Autodesk Inventor part; units mm, degrees
(part 3 of 3)
  arc A872 (130.3995, -26.0356) -> (130.7044, -25.7308) centre (130.3995, -25.7308) ccw
  line L653 (130.3995, -11.9894) -> (116.9629, -11.9894)
  arc A873 (90.4644, -25.7308) -> (90.7692, -26.0356) centre (90.7692, -25.7308) ccw
  arc A874 (90.7692, -11.9894) -> (90.4644, -12.2942) centre (90.7692, -12.2942) ccw
  line L654 (90.4644, -12.2942) -> (90.4644, -25.7308)
  arc A875 (104.5106, -12.2942) -> (104.2058, -11.9894) centre (104.2058, -12.2942) ccw
  line L655 (104.5106, -25.7308) -> (104.5106, -12.2942)
  line L656 (90.7692, -26.0356) -> (104.2058, -26.0356)
  line L657 (90.4644, -26.0356) -> (104.5106, -11.9894) construction
  line L658 (104.5106, -26.0356) -> (90.4644, -11.9894) construction
  arc A876 (104.2058, -26.0356) -> (104.5106, -25.7308) centre (104.2058, -25.7308) ccw
  line L659 (104.2058, -11.9894) -> (90.7692, -11.9894)
  arc A877 (135.7082, -6.6808) -> (136.0129, -6.9856) centre (136.0129, -6.6808) ccw
  arc A878 (136.0129, 7.0606) -> (135.7082, 6.7558) centre (136.0129, 6.7558) ccw
  line L660 (135.7082, 6.7558) -> (135.7082, -6.6808)
  arc A879 (149.7544, 6.7558) -> (149.4495, 7.0606) centre (149.4495, 6.7558) ccw
  line L661 (149.7544, -6.6808) -> (149.7544, 6.7558)
  line L662 (136.0129, -6.9856) -> (149.4495, -6.9856)
  line L663 (135.7082, -6.9856) -> (149.7544, 7.0606) construction
  line L664 (149.7544, -6.9856) -> (135.7082, 7.0606) construction
  arc A880 (149.4495, -6.9856) -> (149.7544, -6.6808) centre (149.4495, -6.6808) ccw
  line L665 (149.4495, 7.0606) -> (136.0129, 7.0606)
  arc A881 (135.7082, 12.3692) -> (136.0129, 12.0644) centre (136.0129, 12.3692) ccw
  arc A882 (136.0129, 26.1106) -> (135.7082, 25.8058) centre (136.0129, 25.8058) ccw
  line L666 (135.7082, 25.8058) -> (135.7082, 12.3692)
  arc A883 (149.7544, 25.8058) -> (149.4495, 26.1106) centre (149.4495, 25.8058) ccw
  line L667 (149.7544, 12.3692) -> (149.7544, 25.8058)
  line L668 (136.0129, 12.0644) -> (149.4495, 12.0644)
  line L669 (135.7082, 12.0644) -> (149.7544, 26.1106) construction
  line L670 (149.7544, 12.0644) -> (135.7082, 26.1106) construction
  arc A884 (149.4495, 12.0644) -> (149.7544, 12.3692) centre (149.4495, 12.3692) ccw
  line L671 (149.4495, 26.1106) -> (136.0129, 26.1106)
  arc A885 (135.7082, 31.4192) -> (136.0129, 31.1144) centre (136.0129, 31.4192) ccw
  arc A886 (136.0129, 45.1606) -> (135.7082, 44.8558) centre (136.0129, 44.8558) ccw
  line L672 (135.7082, 44.8558) -> (135.7082, 31.4192)
  arc A887 (149.7544, 44.8558) -> (149.4495, 45.1606) centre (149.4495, 44.8558) ccw
  line L673 (149.7544, 31.4192) -> (149.7544, 44.8558)
  line L674 (136.0129, 31.1144) -> (149.4495, 31.1144)
  line L675 (135.7082, 31.1144) -> (149.7544, 45.1606) construction
  line L676 (149.7544, 31.1144) -> (135.7082, 45.1606) construction
  arc A888 (149.4495, 31.1144) -> (149.7544, 31.4192) centre (149.4495, 31.4192) ccw
  line L677 (149.4495, 45.1606) -> (136.0129, 45.1606)
  arc A889 (78.5582, 31.4192) -> (78.863, 31.1144) centre (78.863, 31.4192) ccw
  arc A890 (78.863, 45.1606) -> (78.5582, 44.8558) centre (78.863, 44.8558) ccw
  line L678 (78.5582, 44.8558) -> (78.5582, 31.4192)
  arc A891 (92.6044, 44.8558) -> (92.2996, 45.1606) centre (92.2996, 44.8558) ccw
  line L679 (92.6044, 31.4192) -> (92.6044, 44.8558)
  line L680 (78.863, 31.1144) -> (92.2996, 31.1144)
  line L681 (78.5582, 31.1144) -> (92.6044, 45.1606) construction
  line L682 (92.6044, 31.1144) -> (78.5582, 45.1606) construction
  arc A892 (92.2996, 31.1144) -> (92.6044, 31.4192) centre (92.2996, 31.4192) ccw
  line L683 (92.2996, 45.1606) -> (78.863, 45.1606)
  arc A893 (88.0832, 12.3692) -> (88.388, 12.0644) centre (88.388, 12.3692) ccw
  arc A894 (88.388, 26.1106) -> (88.0832, 25.8058) centre (88.388, 25.8058) ccw
  line L684 (88.0832, 25.8058) -> (88.0832, 12.3692)
  arc A895 (102.1294, 25.8058) -> (101.8246, 26.1106) centre (101.8246, 25.8058) ccw
  line L685 (102.1294, 12.3692) -> (102.1294, 25.8058)
  line L686 (88.388, 12.0644) -> (101.8246, 12.0644)
  line L687 (88.0832, 12.0644) -> (102.1294, 26.1106) construction
  line L688 (102.1294, 12.0644) -> (88.0832, 26.1106) construction
  arc A896 (101.8246, 12.0644) -> (102.1294, 12.3692) centre (101.8246, 12.3692) ccw
  line L689 (101.8246, 26.1106) -> (88.388, 26.1106)
  arc A897 (111.8957, 12.3692) -> (112.2004, 12.0644) centre (112.2004, 12.3692) ccw
  arc A898 (112.2004, 26.1106) -> (111.8957, 25.8058) centre (112.2004, 25.8058) ccw
  line L690 (111.8957, 25.8058) -> (111.8957, 12.3692)
  arc A899 (125.9419, 25.8058) -> (125.6371, 26.1106) centre (125.6371, 25.8058) ccw
  line L691 (125.9419, 12.3692) -> (125.9419, 25.8058)
  line L692 (112.2004, 12.0644) -> (125.6371, 12.0644)
  line L693 (111.8957, 12.0644) -> (125.9419, 26.1106) construction
  line L694 (125.9419, 12.0644) -> (111.8957, 26.1106) construction
  arc A900 (125.6371, 12.0644) -> (125.9419, 12.3692) centre (125.6371, 12.3692) ccw
  line L695 (125.6371, 26.1106) -> (112.2004, 26.1106)
  line L696 (-138.1229, -13.7293) -> (-122.5019, -13.7293)
  line L697 (-144.6761, -26.4293) -> (-141.5265, -26.4293)
  line L698 (-141.5265, -25.2101) -> (-139.7231, -25.2101)
  line L699 (-144.6761, -25.2101) -> (-144.6761, -26.4293)
  line L700 (-146.4795, -19.0125) -> (-146.4795, -25.2101)
  line L701 (-139.7231, -24.3211) -> (-139.7231, -13.7293)
  line L702 (-146.4795, -25.2101) -> (-144.6761, -25.2101)
  line L703 (-146.4795, -12.8149) -> (-139.7231, -12.8149)
  line L704 (-139.7231, -12.8149) -> (-146.4795, -25.2101) construction
  line L705 (-146.4795, -12.8149) -> (-139.7231, -25.2101) construction
  line L706 (-139.7231, -25.2101) -> (-139.7231, -24.3211)
  line L707 (-147.4193, -16.0153) -> (-147.4193, -19.0125)
  line L708 (-147.4193, -19.0125) -> (-146.4795, -19.0125)
  line L709 (-146.4795, -16.0153) -> (-147.4193, -16.0153)
  line L710 (-146.4795, -12.8149) -> (-146.4795, -16.0153)
  line L711 (-120.6985, -26.4293) -> (-120.6985, -25.2101)
  line L712 (-120.6985, -25.2101) -> (-122.5019, -25.2101)
  line L713 (-117.5489, -26.4293) -> (-120.6985, -26.4293)
  line L714 (-122.5019, -25.2101) -> (-122.5019, -24.3211)
  line L715 (-141.5265, -26.4293) -> (-141.5265, -25.2101)
  circle A901 centre (-143.0505, -27.2675) radius 1.994
  line L716 (-139.7231, -24.3211) -> (-138.1229, -24.3211)
  circle A902 centre (-119.1745, -27.2675) radius 1.994
  line L717 (-115.7455, -25.2101) -> (-117.5489, -25.2101)
  line L718 (-143.1013, -12.8149) -> (-143.1013, -26.4293)
  line L719 (-117.5489, -25.2101) -> (-117.5489, -26.4293)
  circle A903 centre (-119.1745, -12.0275) radius 1.524
  circle A904 centre (-143.0505, -12.0275) radius 1.524
  line L720 (-138.1229, -24.3211) -> (-122.5019, -24.3211)
  line L721 (-139.7231, -12.8149) -> (-139.7231, -13.7293)
  line L722 (-139.7231, -13.7293) -> (-138.1229, -13.7293)
  arc A905 (-137.8181, -12.0021) -> (-138.1229, -12.3069) centre (-137.8181, -12.3069) ccw
  line L723 (-131.1125, -19.0125) -> (-143.1013, -19.0125)
  line L724 (-131.1125, -12.0021) -> (-131.1125, -26.0229)
  line L725 (-124.1021, -12.0021) -> (-138.1229, -26.0229) construction
  arc A906 (-124.1021, -12.3069) -> (-124.4069, -12.0021) centre (-124.4069, -12.3069) ccw
  arc A907 (-138.1229, -25.7181) -> (-137.8181, -26.0229) centre (-137.8181, -25.7181) ccw
  line L726 (-138.1229, -25.7181) -> (-138.1229, -12.3069)
  line L727 (-124.4069, -26.0229) -> (-137.8181, -26.0229)
  line L728 (-138.1229, -12.0021) -> (-124.1021, -26.0229) construction
  line L729 (-137.8181, -12.0021) -> (-124.4069, -12.0021)
  line L730 (-119.1237, -12.8149) -> (-119.1237, -26.4293)
  line L731 (-115.7455, -19.0125) -> (-115.7455, -25.2101)
  line L732 (-115.7455, -12.8149) -> (-115.7455, -16.0153)
  line L733 (-115.7455, -16.0153) -> (-114.8057, -16.0153)
  line L734 (-114.8057, -16.0153) -> (-114.8057, -19.0125)
  arc A908 (-124.4069, -26.0229) -> (-124.1021, -25.7181) centre (-124.4069, -25.7181) ccw
  line L735 (-124.1021, -12.3069) -> (-124.1021, -25.7181)
  line L736 (-122.5019, -24.3211) -> (-122.5019, -13.7293)
  line L737 (-122.5019, -12.8149) -> (-122.5019, -13.7293)
  line L738 (-131.1125, -19.0125) -> (-119.1237, -19.0125)
  line L739 (-114.8057, -19.0125) -> (-115.7455, -19.0125)
  line L740 (-115.7455, -12.8149) -> (-122.5019, -12.8149)
  line L741 (-115.7455, -12.8149) -> (-122.5019, -25.2101) construction
  line L742 (-122.5019, -12.8149) -> (-115.7455, -25.2101) construction
  line L743 (107.1458, 43.4207) -> (122.7669, 43.4207)
  line L744 (100.5926, 30.7207) -> (103.7422, 30.7207)
  line L745 (103.7422, 31.9399) -> (105.5456, 31.9399)
  line L746 (100.5926, 31.9399) -> (100.5926, 30.7207)
  line L747 (98.7892, 38.1375) -> (98.7892, 31.9399)
  line L748 (105.5456, 32.8289) -> (105.5456, 43.4207)
  line L749 (98.7892, 31.9399) -> (100.5926, 31.9399)
  line L750 (98.7892, 44.3351) -> (105.5456, 44.3351)
  line L751 (105.5456, 44.3351) -> (98.7892, 31.9399) construction
  line L752 (98.7892, 44.3351) -> (105.5456, 31.9399) construction
  line L753 (105.5456, 31.9399) -> (105.5456, 32.8289)
  line L754 (97.8495, 41.1347) -> (97.8495, 38.1375)
  line L755 (97.8495, 38.1375) -> (98.7892, 38.1375)
  line L756 (98.7892, 41.1347) -> (97.8495, 41.1347)
  line L757 (98.7892, 44.3351) -> (98.7892, 41.1347)
  line L758 (124.5702, 30.7207) -> (124.5702, 31.9399)
  line L759 (124.5702, 31.9399) -> (122.7669, 31.9399)
  line L760 (127.7198, 30.7207) -> (124.5702, 30.7207)
  line L761 (122.7669, 31.9399) -> (122.7669, 32.8289)
  line L762 (103.7422, 30.7207) -> (103.7422, 31.9399)
  circle A909 centre (102.2182, 29.8825) radius 1.994
  line L763 (105.5456, 32.8289) -> (107.1458, 32.8289)
  circle A910 centre (126.0942, 29.8825) radius 1.994
  line L764 (129.5232, 31.9399) -> (127.7198, 31.9399)
  line L765 (102.1675, 44.3351) -> (102.1675, 30.7207)
  line L766 (127.7198, 31.9399) -> (127.7198, 30.7207)
  circle A911 centre (126.0942, 45.1225) radius 1.524
  circle A912 centre (102.2182, 45.1225) radius 1.524
  line L767 (107.1458, 32.8289) -> (122.7669, 32.8289)
  line L768 (105.5456, 44.3351) -> (105.5456, 43.4207)
  line L769 (105.5456, 43.4207) -> (107.1458, 43.4207)
  arc A913 (107.4506, 45.1479) -> (107.1458, 44.8431) centre (107.4506, 44.8431) ccw
  line L770 (114.1562, 38.1375) -> (102.1675, 38.1375)
  line L771 (114.1562, 45.1479) -> (114.1562, 31.1271)
  line L772 (121.1666, 45.1479) -> (107.1458, 31.1271) construction
  arc A914 (121.1666, 44.8431) -> (120.8618, 45.1479) centre (120.8618, 44.8431) ccw
  arc A915 (107.1458, 31.4319) -> (107.4506, 31.1271) centre (107.4506, 31.4319) ccw
  line L773 (107.1458, 31.4319) -> (107.1458, 44.8431)
  line L774 (120.8618, 31.1271) -> (107.4506, 31.1271)
  line L775 (107.1458, 45.1479) -> (121.1666, 31.1271) construction
  line L776 (107.4506, 45.1479) -> (120.8618, 45.1479)
  line L777 (126.145, 44.3351) -> (126.145, 30.7207)
  line L778 (129.5232, 38.1375) -> (129.5232, 31.9399)
  line L779 (129.5232, 44.3351) -> (129.5232, 41.1347)
  line L780 (129.5232, 41.1347) -> (130.463, 41.1347)
  line L781 (130.463, 41.1347) -> (130.463, 38.1375)
  arc A916 (120.8618, 31.1271) -> (121.1666, 31.4319) centre (120.8618, 31.4319) ccw
  line L782 (121.1666, 44.8431) -> (121.1666, 31.4319)
  line L783 (122.7669, 32.8289) -> (122.7669, 43.4207)
  line L784 (122.7669, 44.3351) -> (122.7669, 43.4207)
  line L785 (114.1562, 38.1375) -> (126.145, 38.1375)
  line L786 (130.463, 38.1375) -> (129.5232, 38.1375)
  line L787 (129.5232, 44.3351) -> (122.7669, 44.3351)
  line L788 (129.5232, 44.3351) -> (122.7669, 31.9399) construction
  line L789 (122.7669, 44.3351) -> (129.5232, 31.9399) construction
  line L790 (104.7646, 5.3207) -> (120.3856, 5.3207)
  line L791 (98.2114, -7.3793) -> (101.361, -7.3793)
  line L792 (101.361, -6.1601) -> (103.1644, -6.1601)
  line L793 (98.2114, -6.1601) -> (98.2114, -7.3793)
  line L794 (96.408, 0.0375) -> (96.408, -6.1601)
  line L795 (103.1644, -5.2711) -> (103.1644, 5.3207)
  line L796 (96.408, -6.1601) -> (98.2114, -6.1601)
  line L797 (96.408, 6.2351) -> (103.1644, 6.2351)
  line L798 (103.1644, 6.2351) -> (96.408, -6.1601) construction
  line L799 (96.408, 6.2351) -> (103.1644, -6.1601) construction
  line L800 (103.1644, -6.1601) -> (103.1644, -5.2711)
  line L801 (95.4682, 3.0347) -> (95.4682, 0.0375)
  line L802 (95.4682, 0.0375) -> (96.408, 0.0375)
  line L803 (96.408, 3.0347) -> (95.4682, 3.0347)
  line L804 (96.408, 6.2351) -> (96.408, 3.0347)
  line L805 (122.189, -7.3793) -> (122.189, -6.1601)
  line L806 (122.189, -6.1601) -> (120.3856, -6.1601)
  line L807 (125.3386, -7.3793) -> (122.189, -7.3793)
  line L808 (120.3856, -6.1601) -> (120.3856, -5.2711)
  line L809 (101.361, -7.3793) -> (101.361, -6.1601)
  circle A917 centre (99.837, -8.2175) radius 1.994
  line L810 (103.1644, -5.2711) -> (104.7646, -5.2711)
  circle A918 centre (123.713, -8.2175) radius 1.994
  line L811 (127.142, -6.1601) -> (125.3386, -6.1601)
  line L812 (99.7862, 6.2351) -> (99.7862, -7.3793)
  line L813 (125.3386, -6.1601) -> (125.3386, -7.3793)
  circle A919 centre (123.713, 7.0225) radius 1.524
  circle A920 centre (99.837, 7.0225) radius 1.524
  line L814 (104.7646, -5.2711) -> (120.3856, -5.2711)
  line L815 (103.1644, 6.2351) -> (103.1644, 5.3207)
  line L816 (103.1644, 5.3207) -> (104.7646, 5.3207)
  arc A921 (105.0694, 7.0479) -> (104.7646, 6.7431) centre (105.0694, 6.7431) ccw
  line L817 (111.775, 0.0375) -> (99.7862, 0.0375)
  line L818 (111.775, 7.0479) -> (111.775, -6.9729)
  line L819 (118.7854, 7.0479) -> (104.7646, -6.9729) construction
  arc A922 (118.7854, 6.7431) -> (118.4806, 7.0479) centre (118.4806, 6.7431) ccw
  arc A923 (104.7646, -6.6681) -> (105.0694, -6.9729) centre (105.0694, -6.6681) ccw
  line L820 (104.7646, -6.6681) -> (104.7646, 6.7431)
  line L821 (118.4806, -6.9729) -> (105.0694, -6.9729)
  line L822 (104.7646, 7.0479) -> (118.7854, -6.9729) construction
  line L823 (105.0694, 7.0479) -> (118.4806, 7.0479)
  line L824 (123.7638, 6.2351) -> (123.7638, -7.3793)
  line L825 (127.142, 0.0375) -> (127.142, -6.1601)
  line L826 (127.142, 6.2351) -> (127.142, 3.0347)
  line L827 (127.142, 3.0347) -> (128.0818, 3.0347)
  line L828 (128.0818, 3.0347) -> (128.0818, 0.0375)
  arc A924 (118.4806, -6.9729) -> (118.7854, -6.6681) centre (118.4806, -6.6681) ccw
  line L829 (118.7854, 6.7431) -> (118.7854, -6.6681)
  line L830 (120.3856, -5.2711) -> (120.3856, 5.3207)
  line L831 (120.3856, 6.2351) -> (120.3856, 5.3207)
  line L832 (111.775, 0.0375) -> (123.7638, 0.0375)
  line L833 (128.0818, 0.0375) -> (127.142, 0.0375)
  line L834 (127.142, 6.2351) -> (120.3856, 6.2351)
  line L835 (127.142, 6.2351) -> (120.3856, -6.1601) construction
  line L836 (120.3856, 6.2351) -> (127.142, -6.1601) construction
  circle A925 centre (-71.613, -46.3175) radius 1.994
  circle A926 centre (28.463, -31.0775) radius 1.524
  circle A927 centre (28.463, -46.3175) radius 1.994
  circle A928 centre (-71.613, -31.0775) radius 1.524
  line L837 (31.8031, -31.8649) -> (31.8031, -35.0653)
  line L838 (31.8031, -44.2601) -> (29.9997, -44.2601)
  line L839 (29.9997, -44.2601) -> (29.9997, -45.4793)
  line L840 (26.8501, -45.4793) -> (26.8501, -44.2601)
  line L841 (26.8501, -44.2601) -> (25.0467, -44.2601)
  line L842 (25.0467, -44.2601) -> (25.0467, -43.3711)
  line L843 (25.0467, -31.8649) -> (25.0467, -32.7793)
  line L844 (25.0467, -43.3711) -> (25.0467, -32.7793)
  line L845 (29.9997, -45.4793) -> (26.8501, -45.4793)
  line L846 (28.4249, -31.8649) -> (28.4249, -45.4793)
  line L847 (31.8031, -38.0625) -> (31.8031, -44.2601)
  line L848 (32.7429, -38.0625) -> (31.8031, -38.0625)
  line L849 (25.0467, -31.8649) -> (31.8031, -44.2601) construction
  line L850 (31.8031, -35.0653) -> (32.7429, -35.0653)
  line L851 (32.7429, -35.0653) -> (32.7429, -38.0625)
  line L852 (31.8031, -31.8649) -> (25.0467, -44.2601) construction
  line L853 (31.8031, -31.8649) -> (25.0467, -31.8649)
  arc A929 (-14.8694, -45.0729) -> (-14.5646, -44.7681) centre (-14.8694, -44.7681) ccw
  line L854 (25.0467, -35.8125) -> (-21.575, -35.8125)
  line L855 (-21.575, -38.0625) -> (28.4249, -38.0625)
  line L856 (25.0467, -40.3125) -> (-21.575, -40.3125)
  line L857 (-71.5749, -31.8649) -> (-71.5749, -45.4793)
  line L858 (-75.8929, -38.0625) -> (-74.9531, -38.0625)
  line L859 (-64.9489, -38.0625) -> (-64.9489, -35.8125)
  line L860 (-68.1967, -35.8125) -> (-21.575, -35.8125)
  line L861 (-21.575, -38.0625) -> (-71.5749, -38.0625)
  line L862 (-68.1967, -40.3125) -> (-21.575, -40.3125)
  arc A930 (-28.2806, -31.0521) -> (-28.5854, -31.3569) centre (-28.2806, -31.3569) ccw
  arc A931 (-28.5854, -44.7681) -> (-28.2806, -45.0729) centre (-28.2806, -44.7681) ccw
  line L863 (-28.5854, -31.3569) -> (-28.5854, -44.7681)
  line L864 (-14.8694, -31.0521) -> (-28.2806, -31.0521)
  line L865 (-28.5854, -45.0729) -> (-14.5646, -31.0521) construction
  line L866 (-14.5646, -45.0729) -> (-28.5854, -31.0521) construction
  line L867 (-14.5646, -44.7681) -> (-14.5646, -31.3569)
  line L868 (-21.575, -31.0521) -> (-21.575, -45.0729)
  line L869 (-28.2806, -45.0729) -> (-14.8694, -45.0729)
  line L870 (-74.9531, -35.0653) -> (-75.8929, -35.0653)
  arc A932 (-14.5646, -31.3569) -> (-14.8694, -31.0521) centre (-14.8694, -31.3569) ccw
  line L871 (-62.9931, -38.0625) -> (-62.9931, -40.3125)
  line L872 (-68.1967, -43.3711) -> (-68.1967, -32.7793)
  line L873 (-70.0001, -45.4793) -> (-70.0001, -44.2601)
  line L874 (-73.1497, -44.2601) -> (-73.1497, -45.4793)
  line L875 (-73.1497, -45.4793) -> (-70.0001, -45.4793)
  line L876 (-74.9531, -31.8649) -> (-74.9531, -35.0653)
  line L877 (-75.8929, -35.0653) -> (-75.8929, -38.0625)
  line L878 (-70.0001, -44.2601) -> (-68.1967, -44.2601)
  line L879 (-74.9531, -44.2601) -> (-73.1497, -44.2601)
  line L880 (-74.9531, -38.0625) -> (-74.9531, -44.2601)
  line L881 (-68.1967, -31.8649) -> (-68.1967, -32.7793)
  line L882 (-74.9531, -31.8649) -> (-68.1967, -31.8649)
  line L883 (-68.1967, -31.8649) -> (-74.9531, -44.2601) construction
  line L884 (-74.9531, -31.8649) -> (-68.1967, -44.2601) construction
  line L885 (-68.1967, -44.2601) -> (-68.1967, -43.3711)
  point P0 (-159.725, 100.05)
  point P1 (159.725, -87.35)
  point P2 (-135.875, 0.0375)
  point P3 (-109.6813, 0.0375)
  point P4 (-90.6312, 0.0375)
  point P5 (-71.5812, 0.0375)
  point P6 (-52.5313, 0.0375)
  point P7 (-62.0563, -19.0125)
  point P8 (-47.7688, 38.1375)
  point P9 (-33.4812, 0.0375)
  point P10 (-23.9562, -19.0125)
  point P11 (-28.7187, 38.1375)
  point P12 (-19.1937, 19.0875)
  point P13 (-14.4313, 0.0375)
  point P14 (-4.9063, -19.0125)
  point P15 (-9.6688, 38.1375)
  point P16 (-0.1438, 19.0875)
  point P17 (4.6187, 0.0375)
  point P18 (14.1437, -19.0125)
  point P19 (9.3812, 38.1375)
  point P20 (23.6688, 0.0375)
  point P21 (33.1938, -19.0125)
  point P22 (28.4313, 38.1375)
  point P23 (37.9563, 19.0875)
  point P24 (42.7188, 0.0375)
  point P25 (52.2438, -19.0125)
  point P26 (47.4813, 38.1375)
  point P27 (57.0063, 19.0875)
  point P28 (61.7687, 0.0375)
  point P29 (80.8187, 0.0375)
  point P30 (71.2937, -19.0125)
  point P31 (47.4813, -38.0625)
  point P32 (104.6312, -38.0625)
  point P33 (123.6812, -38.0625)
  point P34 (123.6812, -19.0125)
  point P35 (142.7312, 0.0375)
  point P36 (118.9187, 19.0875)
  dimension "d700" = 6.35
  dimension "d701" = 12.7
  dimension "d702" = 6.35
  dimension "d703" = 12.7
  dimension "d704" = 25.4
  dimension "d705" = 12.7
  dimension "d706" = 12.7
  dimension "d707" = 123.9
  dimension "d708" = 12.7
  dimension "d709" = 6.35
  dimension "d710" = 14.0462
  dimension "d711" = 14.0462
  dimension "d712" = 0.3048
  dimension "d713" = 0.3048
  dimension "d714" = 0.3048
  dimension "d715" = 0.3048
  dimension "d716" = 14.0462
  dimension "d717" = 14.0462
  dimension "d718" = 0.3048
  dimension "d719" = 0.3048
  dimension "d720" = 0.3048
  dimension "d721" = 0.3048
  dimension "d722" = 14.0462
  dimension "d723" = 14.0462
  dimension "d724" = 0.3048
  dimension "d725" = 0.3048
  dimension "d726" = 0.3048
  dimension "d727" = 0.3048
  dimension "d728" = 14.0462
  dimension "d729" = 14.0462
  dimension "d730" = 0.3048
  dimension "d731" = 0.3048
  dimension "d732" = 0.3048
  dimension "d733" = 0.3048
  dimension "d734" = 14.0462
  dimension "d735" = 14.0462
  dimension "d736" = 0.3048
  dimension "d737" = 0.3048
  dimension "d738" = 0.3048
  dimension "d739" = 0.3048
  dimension "d740" = 14.0462
  dimension "d741" = 14.0462
  dimension "d742" = 0.3048
  dimension "d743" = 0.3048
  dimension "d744" = 0.3048
  dimension "d745" = 0.3048
  dimension "d746" = 14.0462
  dimension "d747" = 14.0462
  dimension "d748" = 0.3048
  dimension "d749" = 0.3048
  dimension "d750" = 0.3048
  dimension "d751" = 0.3048
  dimension "d752" = 14.0462
  dimension "d753" = 14.0462
  dimension "d754" = 0.3048
  dimension "d755" = 0.3048
  dimension "d756" = 0.3048
  dimension "d757" = 0.3048
  dimension "d758" = 14.0462
  dimension "d759" = 14.0462
  dimension "d760" = 0.3048
  dimension "d761" = 0.3048
  dimension "d762" = 0.3048
  dimension "d763" = 0.3048
  constraints: 1772 end point, 1112 point on circle, 933 centre point, 566 point on line, 552 tangent, 165 midpoint, 138 parallel, 96 perpendicular, 88 horizontal, 74 symmetric about line, 24 vertical, 12 collinear, 3 equal radius, 2 other
  measures "d700" distance of L293.start L293.end
  measures "d701" distance of L292.start L292.end
  measures "d702" distance of L294.start L294.end
  measures "d703" distance of L295.start L295.end
  measures "d704" distance of L296.start L300.end
  measures "d705" distance of L300.end point (-159.725, 100.05)
  measures "d706" distance of L307.end L297.end
  measures "d707" distance of L296.end L297.end
  measures "d708" distance of point (159.725, -87.35) L307.end
  measures "d709" radius of A641
  measures "d710" distance of L315.end L316.end
  measures "d711" distance of L316.start L315.end
  measures "d712" radius of A646
  measures "d713" radius of A647
  measures "d714" radius of A648
  measures "d715" radius of A645
  measures "d716" distance of L321.end L322.end
  measures "d717" distance of L322.start L321.end
  measures "d718" radius of A650
  measures "d719" radius of A651
  measures "d720" radius of A652
  measures "d721" radius of A649
  measures "d722" distance of L327.end L328.end
  measures "d723" distance of L328.start L327.end
  measures "d724" radius of A654
  measures "d725" radius of A655
  measures "d726" radius of A656
  measures "d727" radius of A653
  measures "d728" distance of L333.end L334.end
  measures "d729" distance of L334.start L333.end
  measures "d730" radius of A658
  measures "d731" radius of A659
  measures "d732" radius of A660
  measures "d733" radius of A657
  measures "d734" distance of L339.end L340.end
  measures "d735" distance of L340.start L339.end
  measures "d736" radius of A662
  measures "d737" radius of A663
  measures "d738" radius of A664
  measures "d739" radius of A661
  measures "d740" distance of L345.end L346.end
  measures "d741" distance of L346.start L345.end
  measures "d742" radius of A666
  measures "d743" radius of A667
  measures "d744" radius of A668
  measures "d745" radius of A665
  measures "d746" distance of L351.end L352.end
  measures "d747" distance of L352.start L351.end
  measures "d748" radius of A670
  measures "d749" radius of A671
  measures "d750" radius of A672
  measures "d751" radius of A669
  measures "d752" distance of L357.end L358.end
  measures "d753" distance of L358.start L357.end
  measures "d754" radius of A674
  measures "d755" radius of A675
  measures "d756" radius of A676
  measures "d757" radius of A673
  measures "d758" distance of L363.end L364.end
  measures "d759" distance of L364.start L363.end
  measures "d760" radius of A678
  measures "d761" radius of A679
  measures "d762" radius of A680
  measures "d763" radius of A677
extrude "Plate2" add sketch "Sketch1" along normal blind 3.048 contours A3 L15 L14 L13 L12 L11 L10 L9 A2 L8 L7 A1 L6 L5 L4 L3 L2 A0 L1 L0 | L0 L1 L293 L299 L296 L292 L14 L15 A3 | L1 A0 L2 L3 L4 L5 L6 L295 L298 L299 L293 | L292 L296 L297 L294 L7 L8 A2 L9 L10 L11 L12 L13 L14 | L298 L308 L307 L306 | L300 L301 L302 L296 | L295 L6 A1 L7 L294 L297 L298 | L307 L311 A643 L310 A644 L309 | L303 A641 L304 A642 L305 L301
fold "Fold5" angle 90 bend radius 3.048 thickness 3.048 k factor 0.44 line from (159.725, 0, -74.65) to (-159.725, 0, -74.65) line at bend end moving side (0, 0, -1) folds toward (0, -1, 0)
fold "Fold6" angle 84.148 bend radius 3.048 thickness 3.048 k factor 0.44 line from (-159.725, 0, -61.95) to (159.725, 0, -61.95) line at bend centre moving side (0, 0, -1) folds toward (0, -1, 0)
fold "Fold7" angle 90 bend radius 3.048 thickness 3.048 k factor 0.44 line from (159.725, 0, 87.35) to (-159.725, 0, 87.35) line at bend end moving side (0, 0, 1) folds toward (0, -1, 0)
fold "Fold8" angle 95.852 bend radius 3.048 thickness 3.048 k factor 0.44 line from (159.725, 0, 61.95) to (-159.725, 0, 61.95) line at bend centre moving side (0, 0, 1) folds toward (0, -1, 0)
body "Solid3"
